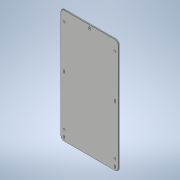
# Autodesk Inventor part: CCU_Fix
Saved by Autodesk Inventor 2021 (Build 250183000, 183)
## iProperties
Created: 2020-10-24
Part Number: CCU_Fix
Material: Generic
Document SubType Name: Modeling
Designer: lgnds
Density: 1 g/cm^3
Appearance: Default
Author: lgnds
Autodesk Inventor part; units mm, degrees
ref_plane "YZ Plane" through (0, 0, 0) normal (1, 0, 0) x (0, 1, 0)
ref_plane "XZ Plane" through (0, 0, 0) normal (0, 1, 0) x (-1, 0, 0)
ref_plane "XY Plane" through (0, 0, 0) normal (0, 0, 1) x (1, 0, 0)
sketch "Sketch1" plane through (0, 0, 0) normal (0, 0, 1) x (1, 0, 0)
  line L0 (-86, -160) -> (86, -160)
  line L1 (86, -160) -> (86, 160)
  line L2 (86, 160) -> (-86, 160)
  line L3 (-86, 160) -> (-86, -160)
  line L4 (-86, -160) -> (86, 160) construction
  line L5 (86, -160) -> (-86, 160) construction
  point P0 (0, 0)
  dimension "d0" = 320
  dimension "d1" = 172
  measures "d0" distance between parallel lines of L0 L2
  measures "d1" distance of L1.end L2.end
extrude "Plate1" add sketch "Sketch1" along normal blind 3.048
sketch "Sketch2" plane through (0, 0, 3.048) normal (0, 0, 1) x (1, 0, 0)
  circle A0 centre (-76, 149) radius 3.25
  line L0 (0, 144.4317) -> (0, -177.0748)
  line L1 (-144.6038, 10) -> (151.531, 10)
  circle A1 centre (76, 149) radius 3.25
  circle A2 centre (-76, -129) radius 3.25
  circle A3 centre (76, -129) radius 3.25
  point P0 (0, 0)
  dimension "d3" = 0
  dimension "d4" = 10
  dimension "d5" = 6.5
  dimension "d6" = 76
  dimension "d7" = 139
  constraints: 4 centre point, 4 end point, 3 symmetric about line, 1 horizontal, 1 vertical, 3 other
  measures "d3" distance from line of point (0, 0) L0
  measures "d4" distance from line of point (0, 0) L1
  measures "d5" diameter of A0
  measures "d6" distance from line of L0 A0.centre
  measures "d7" distance from line of L1 A0.centre
extrude "Cut1" cut sketch "Sketch2" against normal blind 3.048
sketch "Sketch3" plane through (0, 0, 3.048) normal (0, 0, 1) x (1, 0, 0)
  line L0 (-76, -152.5) -> (-76, -147.5) construction
  line L1 (-78.5, -152.5) -> (-78.5, -147.5)
  line L2 (-73.5, -147.5) -> (-73.5, -152.5)
  arc A0 (-78.5, -152.5) -> (-73.5, -152.5) centre (-76, -152.5) ccw
  arc A1 (-73.5, -147.5) -> (-78.5, -147.5) centre (-76, -147.5) ccw
  line L3 (76, -152.5) -> (76, -147.5) construction
  line L4 (73.5, -152.5) -> (73.5, -147.5)
  line L5 (78.5, -147.5) -> (78.5, -152.5)
  arc A2 (73.5, -152.5) -> (78.5, -152.5) centre (76, -152.5) ccw
  arc A3 (78.5, -147.5) -> (73.5, -147.5) centre (76, -147.5) ccw
  line L6 (-23.5, 120) -> (-28.5, 120) construction
  line L7 (-23.5, 122.5) -> (-28.5, 122.5) construction
  line L8 (-28.5, 117.5) -> (-23.5, 117.5) construction
  arc A4 (-23.5, 117.5) -> (-23.5, 122.5) centre (-23.5, 120) ccw construction
  arc A5 (-28.5, 122.5) -> (-28.5, 117.5) centre (-28.5, 120) ccw construction
  line L9 (76, 17.5) -> (76, 22.5) construction
  line L10 (78.5, 17.5) -> (78.5, 22.5)
  line L11 (73.5, 22.5) -> (73.5, 17.5)
  arc A6 (73.5, 17.5) -> (78.5, 17.5) centre (76, 17.5) ccw
  arc A7 (78.5, 22.5) -> (73.5, 22.5) centre (76, 22.5) ccw
  line L12 (86, -160) -> (-86, -160) projected
  line L13 (-86, 160) -> (86, 160) projected
  line L14 (-86, -160) -> (-86, 160) projected
  line L15 (-76, 17.5) -> (-76, 22.5) construction
  line L16 (-78.5, 17.5) -> (-78.5, 22.5)
  line L17 (-73.5, 22.5) -> (-73.5, 17.5)
  arc A8 (-78.5, 17.5) -> (-73.5, 17.5) centre (-76, 17.5) ccw
  arc A9 (-73.5, 22.5) -> (-78.5, 22.5) centre (-76, 22.5) ccw
  line L18 (86, 160) -> (86, -160) projected
  point P0 (0, 0)
  point P1 (-76, -150)
  point P2 (76, -150)
  point P3 (-26, 120)
  point P4 (76, 20)
  point P5 (-76, 20)
  dimension "d12" = 10
  dimension "d13" = 10
  dimension "d14" = 170
  dimension "d16" = 40
  dimension "d17" = 0
  dimension "d18" = 60
  dimension "d19" = 170
  dimension "d20" = 0
  dimension "d21" = 5
  dimension "d22" = 5
  dimension "d23" = 5
  dimension "d24" = 5
  dimension "d25" = 5
  dimension "d26" = 2.5
  dimension "d27" = 2.5
  dimension "d28" = 2.5
  dimension "d29" = 2.5
  dimension "d30" = 2.5
  dimension "d33" = 10
  dimension "d34" = 10
  constraints: 40 end point, 20 point on circle, 20 tangent, 10 centre point, 6 parallel, 5 midpoint, 3 vertical, 1 horizontal
  measures "d12" distance from line of L12 point (-76, -150)
  measures "d13" distance from line of L12 point (76, -150)
  measures "d14" distance of point (76, -150) point (76, 20)
  measures "d16" distance from line of L13 point (-26, 120)
  measures "d17" horizontal distance of point (76, -150) point (76, 20)
  measures "d18" distance from line of L14 point (-26, 120)
  measures "d19" distance of point (-76, -150) point (-76, 20)
  measures "d20" horizontal distance of point (-76, 20) point (-76, -150)
  measures "d21" distance of L17.start L17.end
  measures "d22" distance of L8.start L8.end
  measures "d23" distance of L11.start L11.end
  measures "d24" distance of L2.start L2.end
  measures "d25" distance of L4.start L4.end
  measures "d26" radius of A1
  measures "d27" radius of A3
  measures "d28" radius of A9
  measures "d29" radius of A7
  measures "d30" radius of A5
  measures "d33" distance from line of L14 point (-76, -150)
  measures "d34" distance from line of L18 point (76, -150)
extrude "Cut2" cut sketch "Sketch3" against normal blind 3.048 contours L1 A1 L2 A0 | L4 A3 L5 A2 | A6 L11 A7 L10 | L16 A9 L17 A8
ref_plane "Work Plane1" through (86, 160, 0) normal (0, 0.9659258, -0.258819) x (-1, 0, 0)
fillet "Fillet1" radius 10 2 edges at (-86, -160, 1.524) (86, -160, 1.524)
sketch "Sketch7" plane through (0, 0, 3.048) normal (0, 0, 1) x (1, 0, 0)
  line L0 (86, 160) -> (-86, 160)
  line L1 (-86, 160) -> (86, 160)
  line L2 (86, 160) -> (86, 180)
  line L3 (86, 180) -> (-86, 180)
  line L4 (-86, 180) -> (-86, 160)
  point P0 (0, 0)
  dimension "d50" = 20
  measures "d50" distance between parallel lines of L0 L3
sheet face with bend "Face4" sketch "Sketch7" thickness 3.048 toward (0, 0, -1) bend radius 3.048 relief straight relief width 3.048 relief depth 1.524
bend "Bend3"
sketch "Sketch8" plane through (0, 0, 3.048) normal (0, 0, 1) x (1, 0, 0)
  line L0 (0, 167.5) -> (0, 172.5) construction
  line L1 (2.5, 167.5) -> (2.5, 172.5)
  line L2 (-2.5, 172.5) -> (-2.5, 167.5)
  arc A0 (-2.5, 167.5) -> (2.5, 167.5) centre (0, 167.5) ccw
  arc A1 (2.5, 172.5) -> (-2.5, 172.5) centre (0, 172.5) ccw
  line L3 (86, 180) -> (-86, 180) projected
  line L4 (86, 180) -> (86, -150) projected
  line L5 (-86, 180) -> (-86, -150) projected
  point P0 (0, 0)
  point P1 (0, 170)
  dimension "d56" = 2.5
  dimension "d57" = 5
  dimension "d58" = 10
  dimension "d59" = 172
  dimension "d60" = 86
  constraints: 8 end point, 4 point on circle, 4 tangent, 2 centre point, 1 midpoint, 1 parallel, 1 vertical
  measures "d56" radius of A1
  measures "d57" distance of L2.start L2.end
  measures "d58" distance from line of L3 point (0, 170)
  measures "d59" distance between parallel lines of L4 L5
  measures "d60" distance from line of L5 point (0, 170)
extrude "Cut3" cut sketch "Sketch8" against normal blind 3.048
fillet "Corner Round1" radius 10 2 edges at (86, 180, 1.524) (-86, 180, 1.524)
chamfer "Chamfer1" distance 0.75 angle 45 8 edges at (0, -160, 3.048) (-83.0711, -157.0711, 3.048) (-86, 10, 3.048) (-83.0711, 177.0711, 3.048) (0, 180, 3.048) (83.0711, 177.0711, 3.048) (86, 10, 3.048) (83.0711, -157.0711, 3.048)
equation "\"d12\" = d11"
equation "\"d13\" = d11"
equation "\"d22\" = d21"
equation "\"d23\" = d21"
equation "\"d24\" = d21"
equation "\"d25\" = d21"
equation "\"d27\" = d26"
equation "\"d28\" = d26"
equation "\"d29\" = d28"
equation "\"d30\" = d28"
equation "\"d60\" = 0.5 * d59"
equation "\"BendRadius\" = Thickness"
equation "\"BendReliefWidth\" = Thickness"
equation "\"BendReliefDepth\" = 0.5 * Thickness"
equation "\"CornerReliefSize\" = 4 * Thickness"
equation "\"MinimumRemnant\" = 2 * Thickness"
equation "\"TransitionRadius\" = BendRadius"
equation "\"JacobiRadiusSize\" = BendRadius"
equation "\"GapSize\" = Thickness"
equation "\"d11\" = 10"
body "Solid1"
